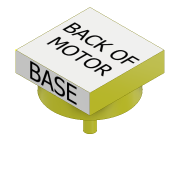
# Autodesk Inventor part: Input Motor
Saved by Autodesk Inventor 2017 (Build 210142000, 142)
## iProperties
Created: 2016-09-28
Part Number: Input Motor
Material: Stainless Steel
Document SubType Name: Modeling
Designer: cmcdona
Density: 8 g/cm^3
Appearance: Yellow
Author: cmcdona
Autodesk Inventor part; units mm, degrees
ref_plane "YZ Plane" through (0, 0, 0) normal (1, 0, 0) x (0, 1, 0)
ref_plane "XZ Plane" through (0, 0, 0) normal (0, 1, 0) x (-1, 0, 0)
ref_plane "XY Plane" through (0, 0, 0) normal (0, 0, 1) x (1, 0, 0)
sketch "Sketch1" plane through (0, 0, 0) normal (0, 0, 1) x (1, 0, 0)
  line L0 (0, 0) -> (15, 0)
  line L1 (15, 0) -> (15, 15)
  line L2 (15, 15) -> (0, 15)
  line L3 (0, 15) -> (0, 0)
  dimension "d0" = 15
  dimension "d1" = 15
  constraints: 8 end point, 2 parallel, 1 horizontal, 1 perpendicular
  measures "d0" distance of L2.end L1.end
  measures "d1" distance of L1.end L0.end
extrude "Extrusion1" add sketch "Sketch1" against normal blind 4
sketch "Sketch2" plane through (0, 0, -4) normal (0, 0, -1) x (-1, 0, 0)
  circle A0 centre (-7.5, 7.5) radius 7.5
  point P0 (0, 0)
  dimension "d4" = 15
  constraints: 1 centre point
  measures "d4" diameter of A0
extrude "Extrusion2" add sketch "Sketch2" along normal blind 3
sketch "Sketch3" plane through (7.5, 7.5, -7) normal (0, 0, -1) x (-1, 0, 0)
  circle A0 centre (0, 0) radius 1
  point P0 (7.5, -7.5)
  dimension "d7" = 2
  constraints: 1 centre point
  measures "d7" diameter of A0
extrude "Extrusion3" add sketch "Sketch3" along normal blind 7
sketch "Sketch4" plane through (0, 0, 0) normal (0, 0, 1) x (1, 0, 0)
  line L0 (0.2915, 14.885) -> (14.8969, 14.885) construction
  line L1 (14.8969, 14.885) -> (14.8969, 0.1242) construction
  line L2 (14.8969, 0.1242) -> (0.2915, 0.1242) construction
  line L3 (0.2915, 0.1242) -> (0.2915, 14.885) construction
  point P0 (0, 0)
  constraints: 2 other
sketch "Sketch5" plane through (0, 0, 0) normal (0, -1, 0) x (1, 0, 0)
  line L0 (0.1529, -0.1223) -> (14.8622, -0.1223) construction
  line L1 (14.8622, -0.1223) -> (14.8622, -3.792) construction
  line L2 (14.8622, -3.792) -> (0.1529, -3.792) construction
  line L3 (0.1529, -3.792) -> (0.1529, -0.1223) construction
  point P0 (0, 0)
  constraints: 2 other
body "Solid1"
